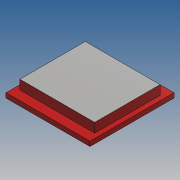
# Autodesk Inventor part: pantalla
Saved by Autodesk Inventor 2017 (Build 210142000, 142)
## iProperties
Part Number: pantalla
Material: Genérico
Document SubType Name: Modeling
Designer: Leo
Density: 1 g/cm^3
Appearance: Rojo
Author: Leo
Autodesk Inventor part; units mm, degrees
ref_plane "YZ Plane" through (0, 0, 0) normal (1, 0, 0) x (0, 1, 0)
ref_plane "XZ Plane" through (0, 0, 0) normal (0, 1, 0) x (-1, 0, 0)
ref_plane "XY Plane" through (0, 0, 0) normal (0, 0, 1) x (1, 0, 0)
sketch "Boceto1" plane through (0, 0, 0) normal (0, 0, 1) x (1, 0, 0)
  line L0 (-22.5, 22.5) -> (22.5, 22.5)
  line L1 (22.5, 22.5) -> (22.5, -22.5)
  line L2 (22.5, -22.5) -> (-22.5, -22.5)
  line L3 (-22.5, -22.5) -> (-22.5, 22.5)
  line L4 (-20, 17.5) -> (20, 17.5)
  line L5 (20, 17.5) -> (20, -17.5)
  line L6 (20, -17.5) -> (-20, -17.5)
  line L7 (-20, -17.5) -> (-20, 17.5)
  point P0 (0, 0)
  point P1 (-22.5, 0)
  point P2 (0, 22.5)
  point P3 (-20, 0)
  point P4 (0, 17.5)
  dimension "d0" = 45
  dimension "d1" = 45
  dimension "d2" = 35
  dimension "d3" = 40
  constraints: 16 end point, 4 midpoint, 4 parallel, 2 horizontal, 2 horizontal alignment, 2 perpendicular, 2 vertical alignment
  measures "d0" distance of L2.end L0.start
  measures "d1" distance of L0.start L0.end
  measures "d2" distance of L4.end L5.end
  measures "d3" distance of L5.end L6.end
extrude "Extrusión1" add sketch "Boceto1" against normal blind 2.5 contours L0 L1 L2 L3 | L4 L5 L6 L7
extrude "Extrusión2" add sketch "Boceto1" along normal blind 5 contours L4 L5 L6 L7
equation "\"d1\" = d0"
